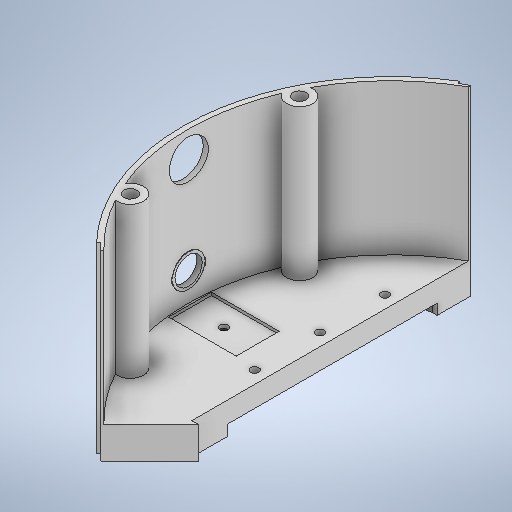
# Autodesk Inventor part: left_hull
Saved by Autodesk Inventor 2025 (Build 290162000, 162)
## iProperties
Created: 2026-03-19
Part Number: left_hull
Material: Generic
Document SubType Name: Modeling
Designer: Luca
Density: 1 g/cm^3
Appearance: Default
Author: Luca
Autodesk Inventor part; units mm, degrees
ref_plane "YZ Plane" through (0, 0, 0) normal (1, 0, 0) x (0, 1, 0)
ref_plane "XZ Plane" through (0, 0, 0) normal (0, 1, 0) x (-1, 0, 0)
ref_plane "XY Plane" through (0, 0, 0) normal (0, 0, 1) x (1, 0, 0)
derived "sk_reservoir.ipt"
sketch "walls" plane through (0, -70, 0) normal (0, 1, 0) x (-1, 0, 0)
  circle A0 centre (0, 0) radius 80
  line L0 (38, -69.4029) -> (38, 38)
  line L1 (38, 38) -> (-69.4029, 38)
  line L2 (35, -68.5857) -> (35, 35)
  line L3 (35, 35) -> (-68.5857, 35)
  arc A1 (-68.5857, 35) -> (35, -68.5857) centre (0, 0) ccw
  arc A2 (38.25, -67.9775) -> (-67.9775, 38.25) centre (0, 0) ccw
  line L4 (80, 0) -> (-80, 0) construction
  line L5 (0, -80) -> (0, 80) construction
  arc A3 (57.0831, 54.4315) -> (54.4315, 57.0831) centre (0, 0) ccw
  line L6 (57.0831, 54.4315) -> (57.8788, 55.2272)
  arc A4 (57.0871, 54.7889) -> (54.427, 57.4322) centre (0, 0) ccw
  line L7 (57.706, 55.4078) -> (57.0871, 54.7889)
  line L8 (38.25, -68.9797) -> (38.25, 38.25)
  line L9 (38.25, 38.25) -> (-68.9797, 38.25)
  line L10 (0, 0) -> (56.5685, 56.5685) construction
  line L11 (54.4315, 57.0831) -> (35.5983, 38.25)
  line L12 (54.427, 57.4322) -> (35.2448, 38.25)
  arc A5 (-67.18, 41.3294) -> (-68.9797, 38.25) centre (0, 0) ccw
  arc A6 (-67.524, 41.2465) -> (-69.4029, 38) centre (0, 0) ccw
  line L13 (-67.18, 41.3294) -> (-68.14, 41.9158)
  line L14 (-67.524, 41.2465) -> (-68.2707, 41.7027)
  arc A7 (38, -69.4029) -> (41.2465, -67.524) centre (0, 0) ccw
  line L15 (41.2465, -67.524) -> (41.7027, -68.2707)
  arc A8 (38.25, -68.9797) -> (41.3294, -67.18) centre (0, 0) ccw
  line L16 (41.3294, -67.18) -> (41.9158, -68.14)
  point P0 (35.8974, -71.4939)
  point P1 (53.8126, 56.4642)
  point P2 (-67.9775, 38.25)
sketch "mount" plane through (0, -70, 0) normal (0, 1, 0) x (-1, 0, 0)
  line L0 (38, -69.4029) -> (38, 38)
  line L1 (38, -55.7015) -> (40, -55.7015)
  arc A0 (40, -55.7015) -> (48, -47.7015) centre (40, -47.7015) ccw
  line L2 (48, -47.7015) -> (48, 16.2985)
  arc A1 (48, 16.2985) -> (40, 24.2985) centre (40, 16.2985) ccw
  line L3 (40, 24.2985) -> (38, 24.2985)
  line L4 (48, -15.7015) -> (38, -15.7015) construction
  line L5 (43, -55.7015) -> (43, 24.2985) construction
  line L6 (38, -55.9515) -> (40, -55.9515)
  line L7 (48.25, -47.7015) -> (48.25, 16.2985)
  line L8 (38, 24.5485) -> (40, 24.5485)
  arc A2 (48.25, 16.2985) -> (40, 24.5485) centre (40, 16.2985) ccw
  arc A3 (40, -55.9515) -> (48.25, -47.7015) centre (40, -47.7015) ccw
  line L9 (38.25, -68.9797) -> (38.25, 38.25)
  circle A4 centre (43, -15.7015) radius 1.6
  line L10 (43, -12.3015) -> (45.9445, -14.0015)
  line L11 (45.9445, -14.0015) -> (45.9445, -17.4015)
  line L12 (45.9445, -17.4015) -> (43, -19.1015)
  line L13 (43, -19.1015) -> (40.0555, -17.4015)
  line L14 (40.0555, -17.4015) -> (40.0555, -14.0015)
  line L15 (40.0555, -14.0015) -> (43, -12.3015)
  line L16 (-119, -119) -> (119, 119) construction
  arc A5 (-47.7015, 48) -> (-55.7015, 40) centre (-47.7015, 40) ccw
  line L17 (-55.7015, 38) -> (-55.7015, 40)
  line L18 (-15.7015, 48) -> (-15.7015, 38) construction
  line L19 (-47.7015, 48) -> (16.2985, 48)
  line L20 (-55.7015, 43) -> (24.2985, 43) construction
  line L21 (-69.4029, 38) -> (38, 38)
  line L22 (24.2985, 40) -> (24.2985, 38)
  arc A6 (24.2985, 40) -> (16.2985, 48) centre (16.2985, 40) ccw
  line L23 (24.5485, 38) -> (24.5485, 40)
  arc A7 (24.5485, 40) -> (16.2985, 48.25) centre (16.2985, 40) ccw
  line L24 (-14.0015, 40.0555) -> (-12.3015, 43)
  line L25 (-12.3015, 43) -> (-14.0015, 45.9445)
  line L26 (-17.4015, 40.0555) -> (-14.0015, 40.0555)
  line L27 (-14.0015, 45.9445) -> (-17.4015, 45.9445)
  circle A8 centre (-15.7015, 43) radius 1.6
  line L28 (-19.1015, 43) -> (-17.4015, 40.0555)
  line L29 (-17.4015, 45.9445) -> (-19.1015, 43)
  line L30 (-47.7015, 48.25) -> (16.2985, 48.25)
  line L31 (-68.9797, 38.25) -> (38.25, 38.25)
  arc A9 (-47.7015, 48.25) -> (-55.9515, 40) centre (-47.7015, 40) ccw
  line L32 (-55.9515, 38) -> (-55.9515, 40)
  point P0 (0, 0)
  point P1 (38.25, -55.9515)
  point P2 (38.25, 24.5485)
sketch "lid_mount" plane through (0, -70, 0) normal (0, 1, 0) x (-1, 0, 0)
  line L0 (35, -68.5857) -> (35, 35) construction
  line L1 (35, 35) -> (-68.5857, 35) construction
  line L2 (38, 38) -> (-69.4029, 38) construction
  line L3 (38, -69.4029) -> (38, 38) construction
  circle A0 centre (32.5, -67.5925) radius 5
  circle A1 centre (-67.5925, 32.5) radius 5
  circle A2 centre (-67.5925, -32.5) radius 5
  circle A3 centre (-32.5, -67.5925) radius 5
  line L4 (-32.5, -67.5925) -> (32.5, -67.5925) construction
  circle A4 centre (0, 0) radius 80
  circle A5 centre (-67.5925, -32.5) radius 2.5
  circle A6 centre (32.5, -67.5925) radius 2.5
  circle A7 centre (-67.5925, 32.5) radius 2.5
  circle A8 centre (-32.5, -67.5925) radius 2.5
  circle A9 centre (67.5925, -32.5) radius 5
  circle A10 centre (-32.5, 67.5925) radius 5
  circle A11 centre (67.5925, -32.5) radius 2.5
  circle A12 centre (-32.5, 67.5925) radius 2.5
  circle A13 centre (32.5, 67.5925) radius 2.5
  circle A14 centre (32.5, 67.5925) radius 5
  circle A15 centre (67.5925, 32.5) radius 2.5
  circle A16 centre (67.5925, 32.5) radius 5
  line L5 (67.5925, 32.5) -> (67.5925, -32.5) construction
  line L6 (32.5, 67.5925) -> (-32.5, 67.5925) construction
  line L7 (0, 67.5925) -> (0, 0)
  line L8 (67.5925, 0) -> (0, 0)
  circle A17 centre (-67.5925, -32.5) radius 2.1
  circle A18 centre (32.5, 67.5925) radius 2.1
  circle A19 centre (67.5925, 32.5) radius 2.1
  circle A20 centre (32.5, -67.5925) radius 2.1
  circle A21 centre (-32.5, -67.5925) radius 2.1
  circle A22 centre (-67.5925, 32.5) radius 2.1
  circle A23 centre (-32.5, 67.5925) radius 2.1
  line L9 (33.7759, 70.2462) -> (34.6667, 72.0987) construction
  circle A24 centre (67.5925, -32.5) radius 2.1
  circle A25 centre (0, 0) radius 1.6
  line L10 (-3.4, 0) -> (-1.7, 2.9445)
  line L11 (-1.7, 2.9445) -> (1.7, 2.9445)
  line L12 (1.7, 2.9445) -> (3.4, 0)
  line L13 (3.4, 0) -> (1.7, -2.9445)
  line L14 (1.7, -2.9445) -> (-1.7, -2.9445)
  line L15 (-1.7, -2.9445) -> (-3.4, 0)
  circle A26 centre (0, 0) radius 5
  circle A27 centre (0, 0) radius 1.35
  line L16 (-67.5925, 32.5) -> (-67.5925, -32.5) construction
  point P0 (0, -67.5925)
  point P1 (-67.5925, 0)
ref_plane "bottom_plane" through (0, -70, 0) normal (0, 1, 0) x (-1, 0, 0)
ref_plane "hull_hole_top" through (0, -65.9, 0) normal (0, 1, 0) x (-1, 0, 0)
ref_plane "hull_mount_top" through (0, -57.9, 0) normal (0, 1, 0) x (-1, 0, 0)
ref_plane "mount_nut_center" through (0, -61.9, 0) normal (0, 1, 0) x (-1, 0, 0)
sketch "button_1" plane through (-80, 0, 0) normal (1, 0, 0) x (0, 1, 0)
  line L0 (-57.9, 133.17) -> (-57.9, -125.8542)
  line L1 (-43.8, -4) -> (-49.9, -4)
  line L2 (-49.9, -4) -> (-49.9, 4)
  line L3 (-49.9, 4) -> (-43.8, 4)
  line L4 (-43.8, 4) -> (-43.8, -4)
  line L5 (-43.8, -1.25) -> (-49.9, -1.25)
  line L6 (-49.9, -1.25) -> (-49.9, 1.25)
  line L7 (-49.9, 1.25) -> (-43.8, 1.25)
  line L8 (-43.8, 1.25) -> (-43.8, -1.25)
  line L9 (-49.9, 0) -> (-0.1295, 0) construction
  line L10 (-132, 0) -> (302, 0) construction
  circle A0 centre (-46.85, 0) radius 6.5
  circle A1 centre (-46.85, 0) radius 6.25
  circle A2 centre (-46.85, 0) radius 5.25
  circle A3 centre (-46.85, 0) radius 5
  circle A4 centre (-46.85, 0) radius 8
  line L11 (-46.85, -8) -> (-57.9, -8)
  line L12 (-46.85, 8) -> (-57.9, 8)
  point P0 (0, 0)
  point P1 (-46.85, 4)
  point P2 (-43.8, 1.25)
ref_plane "button_stop" through (-77.75, 0, 0) normal (1, 0, 0) x (0, 1, 0)
sketch "button_mount" plane through (0, -57.9, 0) normal (0, 1, 0) x (-1, 0, 0)
  line L0 (80, 133.17) -> (80, -125.8542)
  line L1 (77.5, -148.4939) -> (77.5, 153.4424)
  line L2 (74.2, -8) -> (54.2, -8)
  line L3 (54.2, -8) -> (54.2, 8)
  line L4 (54.2, 8) -> (74.2, 8)
  line L5 (74.2, 8) -> (74.2, -8)
  circle A0 centre (61.2, 0) radius 1.6 construction
  line L6 (77.2, -8.25) -> (51.2, -8.25)
  line L7 (51.2, -8.25) -> (51.2, 8.25)
  line L8 (51.2, 8.25) -> (77.2, 8.25)
  line L9 (77.2, 8.25) -> (77.2, -8.25)
  circle A1 centre (64.2, 0) radius 1.6
  arc A2 (61.2, 1.6) -> (61.2, -1.6) centre (61.2, 0) ccw
  circle A3 centre (67.2, 0) radius 1.6 construction
  line L10 (61.2, -1.6) -> (67.2, -1.6)
  line L11 (61.2, 1.6) -> (67.2, 1.6)
  arc A4 (67.2, -1.6) -> (67.2, 1.6) centre (67.2, 0) ccw
  line L12 (60.8, 0) -> (62.5, 2.9445)
  line L13 (62.5, 2.9445) -> (65.9, 2.9445)
  line L14 (65.9, 2.9445) -> (67.6, 0)
  line L15 (67.6, 0) -> (65.9, -2.9445)
  line L16 (65.9, -2.9445) -> (62.5, -2.9445)
  line L17 (62.5, -2.9445) -> (60.8, 0)
  point P0 (0, 0)
  point P1 (80, -8)
  point P2 (80, -8)
  point P3 (80, -8)
  point P4 (80, 8)
  point P5 (80, 8)
  point P6 (80, 8)
  point P7 (54.2, 0)
sketch "pipe_out" plane through (-77.5, 0, 0) normal (1, 0, 0) x (0, 1, 0)
  line L0 (-132, 0) -> (302, 0)
  circle A0 centre (-10, 0) radius 7.5
  line L1 (0, 153.4424) -> (0, -148.4939)
  circle A1 centre (-10, 0) radius 7.25
  circle A2 centre (-10, 0) radius 5
  circle A3 centre (-10, 0) radius 9.5
  circle A4 centre (-10, 0) radius 6
  circle A5 centre (-10, 0) radius 6.25
  point P0 (0, 0)
  point P1 (-2.5, 0)
  point P2 (-2.75, 0)
extrude "Extrusion1" add sketch "walls" along normal up to surface (12.1 mm away) from surface at 0 contours A0 L16 A8 L8 A2 L11 A3 L6 | A2 L8 L9 L11
extrude "Extrusion2" add sketch "walls" along normal up to surface (70 mm away) from surface at 0 contours A0 L16 A8 L8 A2 L11 A3 L6
extrude "Extrusion3" cut sketch "mount" along normal up to surface (4.1 mm away) from surface at 0 contours L9 L1 A0 L2 A1 L3 L8 A2 L7 A3 L6 | L9 L3 A1 L2 A0 L1 | A4 | L10 L11 L12 L13 L14 L15
extrude "Extrusion4" cut sketch "mount" along normal through all both and the other way through all contours A4
extrude "Extrusion5" cut sketch "mount" along normal mid plane 3 from surface at 8.1 contours A4 | L10 L11 L12 L13 L14 L15
pattern_linear "Rectangular Pattern1" count 2 spacing 25 along (0, 0, 1) of "Extrusion4", "Extrusion5"
pattern_linear "Rectangular Pattern2" count 2 spacing 25 along (0, 0, -1) of "Extrusion4", "Extrusion5"
extrude "Extrusion21" cut sketch "button_1" along normal blind 10 from surface at 2.25 contours L1 A3 L4 | A3 L1 | L1 A3 L2 L5 L4 | L4 A3 | L1 L2 A3 | L5 L2 L7 L4 | A3 L2 | L7 L2 A3 L3 L4 | A3 L3 L4 | L2 L3 A3 | L3 A3 | A0 | A1 | A2
extrude "Extrusion18" add sketch "button_1" against normal blind 2 from surface at 2.25 contours L1 A3 L4 | A3 L1 | L1 A3 L2 L5 L4 | L4 A3 | L1 L2 A3 | L5 L2 L7 L4 | A3 L2 | L7 L2 A3 L3 L4 | A3 L3 L4 | L2 L3 A3 | L3 A3 | A1 | A2
extrude "Extrusion12" cut sketch "button_1" along normal through all both and the other way through all contours L1 A3 L4 | A3 L1 | L1 A3 L2 L5 L4 | L4 A3 | L1 L2 A3 | L5 L2 L7 L4 | A3 L2 | L7 L2 A3 L3 L4 | A3 L3 L4 | L2 L3 A3 | L3 A3 | A2
extrude "Extrusion26" add sketch "lid_mount" along normal up to surface (70 mm away) from surface at 0 contours A9 | A16 | A11 | A15 | A19 | A24
extrude "Extrusion27" cut sketch "lid_mount" against normal blind 20 from surface at 70 contours A11 | A15 | A19 | A24
extrude "Extrusion32" cut sketch "button_mount" along normal mid plane 3 from surface at -4 contours A1 | A1 L11 L14 L15 L10 | A1 L10 L17 L12 L11 | L11 L12 L13 L14 | L10 L15 L16 L17
extrude "Extrusion30" cut sketch "button_mount" against normal blind 10 contours A1
extrude "Extrusion31" cut sketch "button_mount" against normal blind 1.1 contours L2 L3 L4 L5 | L6 L7 L8 L9 | A1 | A1 L11 L14 L15 L10 | A1 L10 L17 L12 L11 | L11 L12 L13 L14 | L10 L15 L16 L17 | L12 L17 L10 A2 L11 | L11 A4 L10 L15 L14
extrude "Extrusion33" cut sketch "pipe_out" against normal through all contours A2 L0 A4 | A2 L0 | L0 A2 | L0 A4 A2 | A4 L0 A5 | L0 A5 A4 | A5 L0 A1 | L0 A1 A5 | A1 L0 A0 | L0 A0 A1
body "Solid1"
